Autodesk Fusion 360 part; units mm, degrees
(part 4 of 6)
sketch "mock keys" plane through (0, 0, 0) normal (0, -1, 0) x (1, 0, 0)
  line L0 (140.1031, 86.5919) -> (126.1031, 86.5919)
  line L1 (126.1031, 86.5919) -> (126.1031, 100.5919)
  line L2 (126.1031, 100.5919) -> (140.1031, 100.5919)
  line L3 (140.1031, 100.5919) -> (140.1031, 86.5919)
  line L4 (30.8531, 93.7533) -> (30.8531, 107.7533)
  line L5 (30.8531, 107.7533) -> (44.8531, 107.7533)
  line L6 (44.8531, 107.7533) -> (44.8531, 93.7533)
  line L7 (44.8531, 93.7533) -> (30.8531, 93.7533)
  line L8 (126.1031, 67.5419) -> (126.1031, 81.5419)
  line L9 (126.1031, 81.5419) -> (140.1031, 81.5419)
  line L10 (140.1031, 81.5419) -> (140.1031, 67.5419)
  line L11 (140.1031, 67.5419) -> (126.1031, 67.5419)
  line L12 (49.9031, 98.5158) -> (49.9031, 112.5158)
  line L13 (49.9031, 112.5158) -> (63.9031, 112.5158)
  line L14 (63.9031, 112.5158) -> (63.9031, 98.5158)
  line L15 (63.9031, 98.5158) -> (49.9031, 98.5158)
  line L16 (107.0531, 96.1169) -> (107.0531, 110.1169)
  line L17 (107.0531, 110.1169) -> (121.0531, 110.1169)
  line L18 (121.0531, 110.1169) -> (121.0531, 96.1169)
  line L19 (121.0531, 96.1169) -> (107.0531, 96.1169)
  line L20 (11.8031, 93.7533) -> (11.8031, 107.7533)
  line L21 (11.8031, 107.7533) -> (25.8031, 107.7533)
  line L22 (25.8031, 107.7533) -> (25.8031, 93.7533)
  line L23 (25.8031, 93.7533) -> (11.8031, 93.7533)
  line L24 (49.9031, 41.3658) -> (49.9031, 55.3658)
  line L25 (49.9031, 55.3658) -> (63.9031, 55.3658)
  line L26 (63.9031, 55.3658) -> (63.9031, 41.3658)
  line L27 (63.9031, 41.3658) -> (49.9031, 41.3658)
  line L28 (30.8531, 74.7033) -> (30.8531, 88.7033)
  line L29 (30.8531, 88.7033) -> (44.8531, 88.7033)
  line L30 (44.8531, 88.7033) -> (44.8531, 74.7033)
  line L31 (44.8531, 74.7033) -> (30.8531, 74.7033)
  line L32 (30.8531, 55.6533) -> (30.8531, 69.6533)
  line L33 (30.8531, 69.6533) -> (44.8531, 69.6533)
  line L34 (44.8531, 69.6533) -> (44.8531, 55.6533)
  line L35 (44.8531, 55.6533) -> (30.8531, 55.6533)
  line L36 (11.8031, 17.5533) -> (11.8031, 31.5533)
  line L37 (11.8031, 31.5533) -> (25.8031, 31.5533)
  line L38 (25.8031, 31.5533) -> (25.8031, 17.5533)
  line L39 (25.8031, 17.5533) -> (11.8031, 17.5533)
  line L40 (116.8975, 10.2287) -> (104.7731, 17.2287)
  line L41 (104.7731, 17.2287) -> (106.7731, 20.6928)
  line L42 (106.7731, 20.6928) -> (104.9761, 21.7303)
  line L43 (104.9761, 21.7303) -> (103.3761, 18.959)
  line L44 (103.3761, 18.959) -> (98.3098, 21.884)
  line L45 (98.3098, 21.884) -> (104.5098, 32.6227)
  line L46 (104.5098, 32.6227) -> (109.5761, 29.6977)
  line L47 (109.5761, 29.6977) -> (107.9761, 26.9264)
  line L48 (107.9761, 26.9264) -> (109.7731, 25.8889)
  line L49 (109.7731, 25.8889) -> (111.7731, 29.353)
  line L50 (111.7731, 29.353) -> (123.8975, 22.353)
  line L51 (123.8975, 22.353) -> (121.8975, 18.8889)
  line L52 (121.8975, 18.8889) -> (123.6945, 17.8514)
  line L53 (123.6945, 17.8514) -> (125.2945, 20.6227)
  line L54 (125.2945, 20.6227) -> (130.3607, 17.6977)
  line L55 (130.3607, 17.6977) -> (124.1607, 6.959)
  line L56 (124.1607, 6.959) -> (119.0945, 9.884)
  line L57 (119.0945, 9.884) -> (120.6945, 12.6553)
  line L58 (120.6945, 12.6553) -> (118.8975, 13.6928)
  line L59 (118.8975, 13.6928) -> (116.8975, 10.2287)
  line L60 (30.8531, 36.6033) -> (30.8531, 50.6033)
  line L61 (30.8531, 50.6033) -> (44.8531, 50.6033)
  line L62 (44.8531, 50.6033) -> (44.8531, 36.6033)
  line L63 (44.8531, 36.6033) -> (30.8531, 36.6033)
  line L64 (11.8031, 36.6033) -> (11.8031, 50.6033)
  line L65 (11.8031, 50.6033) -> (25.8031, 50.6033)
  line L66 (25.8031, 50.6033) -> (25.8031, 36.6033)
  line L67 (25.8031, 36.6033) -> (11.8031, 36.6033)
  line L68 (11.8031, 55.6533) -> (11.8031, 69.6533)
  line L69 (11.8031, 69.6533) -> (25.8031, 69.6533)
  line L70 (25.8031, 69.6533) -> (25.8031, 55.6533)
  line L71 (25.8031, 55.6533) -> (11.8031, 55.6533)
  line L72 (11.8031, 74.7033) -> (11.8031, 88.7033)
  line L73 (11.8031, 88.7033) -> (25.8031, 88.7033)
  line L74 (25.8031, 88.7033) -> (25.8031, 74.7033)
  line L75 (25.8031, 74.7033) -> (11.8031, 74.7033)
  line L76 (134.7127, 21.9762) -> (122.5884, 28.9762)
  line L77 (122.5884, 28.9762) -> (129.5884, 41.1005)
  line L78 (129.5884, 41.1005) -> (141.7127, 34.1005)
  line L79 (141.7127, 34.1005) -> (134.7127, 21.9762)
  line L80 (141.6977, -4.0941) -> (129.5734, 2.9059)
  line L81 (129.5734, 2.9059) -> (136.5734, 15.0302)
  line L82 (136.5734, 15.0302) -> (148.6977, 8.0302)
  line L83 (148.6977, 8.0302) -> (141.6977, -4.0941)
  line L84 (30.8531, 17.5533) -> (30.8531, 31.5533)
  line L85 (30.8531, 31.5533) -> (44.8531, 31.5533)
  line L86 (44.8531, 31.5533) -> (44.8531, 17.5533)
  line L87 (44.8531, 17.5533) -> (30.8531, 17.5533)
  line L88 (49.9031, 22.3158) -> (49.9031, 36.3158)
  line L89 (49.9031, 36.3158) -> (63.9031, 36.3158)
  line L90 (63.9031, 36.3158) -> (63.9031, 22.3158)
  line L91 (63.9031, 22.3158) -> (49.9031, 22.3158)
  line L92 (68.9531, 100.8794) -> (68.9531, 114.8794)
  line L93 (68.9531, 114.8794) -> (82.9531, 114.8794)
  line L94 (82.9531, 114.8794) -> (82.9531, 100.8794)
  line L95 (82.9531, 100.8794) -> (68.9531, 100.8794)
  line L96 (68.9531, 81.8294) -> (68.9531, 95.8294)
  line L97 (68.9531, 95.8294) -> (82.9531, 95.8294)
  line L98 (82.9531, 95.8294) -> (82.9531, 81.8294)
  line L99 (82.9531, 81.8294) -> (68.9531, 81.8294)
  line L100 (68.9531, 62.7794) -> (68.9531, 76.7794)
  line L101 (68.9531, 76.7794) -> (82.9531, 76.7794)
  line L102 (82.9531, 76.7794) -> (82.9531, 62.7794)
  line L103 (82.9531, 62.7794) -> (68.9531, 62.7794)
  line L104 (68.9531, 43.7294) -> (68.9531, 57.7294)
  line L105 (68.9531, 57.7294) -> (82.9531, 57.7294)
  line L106 (82.9531, 57.7294) -> (82.9531, 43.7294)
  line L107 (82.9531, 43.7294) -> (68.9531, 43.7294)
  line L108 (76.5731, 22.3158) -> (76.5731, 36.3158)
  line L109 (76.5731, 36.3158) -> (90.5731, 36.3158)
  line L110 (90.5731, 36.3158) -> (90.5731, 22.3158)
  line L111 (90.5731, 22.3158) -> (76.5731, 22.3158)
  line L112 (49.9031, 60.4158) -> (49.9031, 74.4158)
  line L113 (49.9031, 74.4158) -> (63.9031, 74.4158)
  line L114 (63.9031, 74.4158) -> (63.9031, 60.4158)
  line L115 (63.9031, 60.4158) -> (49.9031, 60.4158)
  line L116 (49.9031, 79.4658) -> (49.9031, 93.4658)
  line L117 (49.9031, 93.4658) -> (63.9031, 93.4658)
  line L118 (63.9031, 93.4658) -> (63.9031, 79.4658)
  line L119 (63.9031, 79.4658) -> (49.9031, 79.4658)
  line L120 (126.1031, 48.4919) -> (126.1031, 62.4919)
  line L121 (126.1031, 62.4919) -> (140.1031, 62.4919)
  line L122 (140.1031, 62.4919) -> (140.1031, 48.4919)
  line L123 (140.1031, 48.4919) -> (126.1031, 48.4919)
  line L124 (88.0031, 60.4158) -> (88.0031, 74.4158)
  line L125 (88.0031, 74.4158) -> (102.0031, 74.4158)
  line L126 (102.0031, 74.4158) -> (102.0031, 60.4158)
  line L127 (102.0031, 60.4158) -> (88.0031, 60.4158)
  line L128 (107.0531, 91.0669) -> (121.0531, 91.0669)
  line L129 (121.0531, 91.0669) -> (121.0531, 77.0669)
  line L130 (121.0531, 77.0669) -> (107.0531, 77.0669)
  line L131 (107.0531, 77.0669) -> (107.0531, 91.0669)
  line L132 (88.0031, 79.4658) -> (88.0031, 93.4658)
  line L133 (88.0031, 93.4658) -> (102.0031, 93.4658)
  line L134 (102.0031, 93.4658) -> (102.0031, 79.4658)
  line L135 (102.0031, 79.4658) -> (88.0031, 79.4658)
  line L136 (107.0531, 58.0169) -> (107.0531, 72.0169)
  line L137 (107.0531, 72.0169) -> (121.0531, 72.0169)
  line L138 (121.0531, 72.0169) -> (121.0531, 58.0169)
  line L139 (121.0531, 58.0169) -> (107.0531, 58.0169)
  line L140 (107.0531, 38.9669) -> (107.0531, 52.9669)
  line L141 (107.0531, 52.9669) -> (121.0531, 52.9669)
  line L142 (121.0531, 52.9669) -> (121.0531, 38.9669)
  line L143 (121.0531, 38.9669) -> (107.0531, 38.9669)
  line L144 (88.0031, 41.3658) -> (88.0031, 55.3658)
  line L145 (88.0031, 55.3658) -> (102.0031, 55.3658)
  line L146 (102.0031, 55.3658) -> (102.0031, 41.3658)
  line L147 (102.0031, 41.3658) -> (88.0031, 41.3658)
  circle A0 centre (71.0494, 18.8031) radius 1.1
  line L148 (102.0031, 112.5158) -> (102.0031, 98.5158)
  line L149 (102.0031, 98.5158) -> (88.0031, 98.5158)
  line L150 (88.0031, 98.5158) -> (88.0031, 112.5158)
  line L151 (88.0031, 112.5158) -> (102.0031, 112.5158)
  circle A1 centre (18.8031, 34.0783) radius 1.1
  circle A2 centre (28.3281, 91.2283) radius 1.1
  circle A3 centre (95.25, 34.2547) radius 1.1
  circle A4 centre (115.7464, 33.7256) radius 1.1
  circle A5 centre (146.7556, 76.7997) radius 1.1
  circle A6 centre (157.6917, 44.4147) radius 1.1
  circle A7 centre (146.7556, 37.8883) radius 1.1
  line L152 (151.2227, 12.4159) -> (139.0984, 19.4159)
  line L153 (139.0984, 19.4159) -> (146.0984, 31.5402)
  line L154 (146.0984, 31.5402) -> (158.2227, 24.5402)
  line L155 (158.2227, 24.5402) -> (151.2227, 12.4159)
  circle A8 centre (123.5781, 102.5878) radius 1.1
  circle A9 centre (66.4281, 78.105) radius 1.1
  circle A10 centre (130.9158, 10.2658) radius 1.1
  arc A11 (142.7339, 99.2011) -> (138.7122, 103.2228) centre (138.7122, 99.2011) ccw
  line L156 (138.7122, 103.2228) -> (132.5162, 103.2228)
  arc A12 (131.5417, 103.3426) -> (132.5162, 103.2228) centre (132.5162, 107.2444) ccw
  line L157 (131.5417, 103.3426) -> (126.6957, 104.553)
  arc A13 (123.6486, 108.4548) -> (126.6957, 104.553) centre (127.6703, 108.4548) ccw
  line L158 (123.6486, 108.4548) -> (123.6486, 112.6772)
  line L159 (123.6486, 112.6772) -> (84.9842, 117.4397)
  line L160 (84.9842, 117.4397) -> (66.9572, 117.4397)
  line L161 (66.9572, 117.4397) -> (9.2428, 110.3136)
  line L162 (9.2428, 110.3136) -> (9.2428, 14.9931)
  line L163 (9.2428, 14.9931) -> (103.8578, 14.9931)
  line L164 (103.8578, 14.9931) -> (142.6281, -7.5847)
  line L165 (142.6281, -7.5847) -> (161.7839, 25.5411)
  line L166 (161.7839, 25.5411) -> (152.8134, 30.7285)
  arc A14 (150.7772, 34.2581) -> (152.8134, 30.7285) centre (154.8544, 34.2581) ccw
  line L167 (150.7772, 34.2581) -> (150.7772, 36.2632)
  arc A15 (154.8573, 40.3375) -> (150.7772, 36.2632) centre (154.8544, 36.2603) ccw
  line L168 (154.8573, 40.3375) -> (157.6917, 40.3375)
  arc A16 (157.6917, 40.3375) -> (157.6917, 48.4919) centre (157.6917, 44.4147) ccw
  line L169 (157.6917, 48.4919) -> (146.8111, 48.4919)
  arc A17 (142.7339, 52.5692) -> (146.8111, 48.4919) centre (146.8111, 52.5692) ccw
  line L170 (142.7339, 52.5692) -> (142.7339, 68.7564)
  arc A18 (146.7556, 72.7781) -> (142.7339, 68.7564) centre (146.7556, 68.7564) ccw
  arc A19 (146.7556, 72.7781) -> (146.7556, 80.8214) centre (146.7556, 76.7997) ccw
  arc A20 (142.7339, 84.843) -> (146.7556, 80.8214) centre (146.7556, 84.843) ccw
  line L171 (142.7339, 84.843) -> (142.7339, 99.2011)
  line L172 (9.8031, 71.6533) -> (27.8031, 71.6533)
  line L173 (27.8031, 71.6533) -> (27.8031, 53.6533)
  line L174 (27.8031, 53.6533) -> (9.8031, 53.6533)
  line L175 (9.8031, 53.6533) -> (9.8031, 71.6533)
  line L176 (9.8031, 91.7533) -> (9.8031, 109.7533)
  line L177 (27.8031, 91.7533) -> (9.8031, 91.7533)
  line L178 (9.8031, 109.7533) -> (27.8031, 109.7533)
  line L179 (27.8031, 109.7533) -> (27.8031, 91.7533)
  line L180 (9.8031, 15.5533) -> (9.8031, 33.5533)
  line L181 (27.8031, 15.5533) -> (9.8031, 15.5533)
  line L182 (9.8031, 33.5533) -> (27.8031, 33.5533)
  line L183 (27.8031, 33.5533) -> (27.8031, 15.5533)
  line L184 (9.8031, 34.6033) -> (9.8031, 52.6033)
  line L185 (27.8031, 34.6033) -> (9.8031, 34.6033)
  line L186 (9.8031, 52.6033) -> (27.8031, 52.6033)
  line L187 (27.8031, 52.6033) -> (27.8031, 34.6033)
  line L188 (124.1031, 84.5919) -> (124.1031, 102.5919)
  line L189 (142.1031, 84.5919) -> (124.1031, 84.5919)
  line L190 (124.1031, 102.5919) -> (142.1031, 102.5919)
  line L191 (142.1031, 102.5919) -> (142.1031, 84.5919)
  line L192 (124.1031, 65.5419) -> (124.1031, 83.5419)
  line L193 (142.1031, 65.5419) -> (124.1031, 65.5419)
  line L194 (124.1031, 83.5419) -> (142.1031, 83.5419)
  line L195 (142.1031, 83.5419) -> (142.1031, 65.5419)
  line L196 (124.1031, 46.4919) -> (124.1031, 64.4919)
  line L197 (142.1031, 46.4919) -> (124.1031, 46.4919)
  line L198 (124.1031, 64.4919) -> (142.1031, 64.4919)
  line L199 (142.1031, 64.4919) -> (142.1031, 46.4919)
  line L200 (9.8031, 72.7033) -> (9.8031, 90.7033)
  line L201 (27.8031, 72.7033) -> (9.8031, 72.7033)
  line L202 (9.8031, 90.7033) -> (27.8031, 90.7033)
  line L203 (27.8031, 90.7033) -> (27.8031, 72.7033)
  line L204 (25.8031, 17.5533) -> (25.8031, 31.5533)
  line L205 (11.8031, 31.5533) -> (11.8031, 17.5533)
  line L206 (25.8031, 31.5533) -> (11.8031, 31.5533)
  line L207 (11.8031, 17.5533) -> (25.8031, 17.5533)
  line L208 (30.8531, 17.5533) -> (44.8531, 17.5533)
  line L209 (30.8531, 31.5533) -> (30.8531, 17.5533)
  line L210 (44.8531, 31.5533) -> (30.8531, 31.5533)
  line L211 (44.8531, 17.5533) -> (44.8531, 31.5533)
  line L212 (90.3624, 253.2917) -> (90.3624, 271.2917)
  line L213 (90.3624, 195.0917) -> (108.3624, 195.0917)
  line L214 (90.3624, 252.2417) -> (108.3624, 252.2417)
  line L215 (108.3624, 214.1417) -> (108.3624, 196.1417)
  line L216 (90.3624, 215.1917) -> (90.3624, 233.1917)
  line L217 (108.3624, 196.1417) -> (90.3624, 196.1417)
  line L218 (90.3624, 214.1417) -> (108.3624, 214.1417)
  line L219 (90.3624, 177.0917) -> (90.3624, 195.0917)
  line L220 (108.3624, 234.2417) -> (90.3624, 234.2417)
  line L221 (108.3624, 271.2917) -> (108.3624, 253.2917)
  line L222 (108.3624, 215.1917) -> (90.3624, 215.1917)
  line L223 (108.3624, 253.2917) -> (90.3624, 253.2917)
  line L224 (90.3624, 234.2417) -> (90.3624, 252.2417)
  line L225 (90.3624, 196.1417) -> (90.3624, 214.1417)
  line L226 (108.3624, 233.1917) -> (108.3624, 215.1917)
  line L227 (90.3624, 271.2917) -> (108.3624, 271.2917)
  line L228 (108.3624, 177.0917) -> (90.3624, 177.0917)
  line L229 (90.3624, 233.1917) -> (108.3624, 233.1917)
  line L230 (108.3624, 252.2417) -> (108.3624, 234.2417)
  line L231 (108.3624, 195.0917) -> (108.3624, 177.0917)
  line L232 (90.3624, 195.0917) -> (108.3624, 195.0917)
  line L233 (90.3624, 177.0917) -> (90.3624, 195.0917)
  line L234 (108.3624, 195.0917) -> (108.3624, 177.0917)
  line L235 (108.3624, 252.2417) -> (108.3624, 234.2417)
  line L236 (108.3624, 214.1417) -> (108.3624, 196.1417)
  line L237 (90.3624, 253.2917) -> (90.3624, 271.2917)
  line L238 (90.3624, 196.1417) -> (90.3624, 214.1417)
  line L239 (90.3624, 215.1917) -> (90.3624, 233.1917)
  line L240 (108.3624, 233.1917) -> (108.3624, 215.1917)
  line L241 (108.3624, 271.2917) -> (108.3624, 253.2917)
  line L242 (90.3624, 234.2417) -> (90.3624, 252.2417)
  line L243 (90.3624, 233.1917) -> (108.3624, 233.1917)
  line L244 (108.3624, 253.2917) -> (90.3624, 253.2917)
  line L245 (90.3624, 214.1417) -> (108.3624, 214.1417)
  line L246 (108.3624, 177.0917) -> (90.3624, 177.0917)
  line L247 (108.3624, 215.1917) -> (90.3624, 215.1917)
  line L248 (90.3624, 252.2417) -> (108.3624, 252.2417)
  line L249 (108.3624, 234.2417) -> (90.3624, 234.2417)
  line L250 (108.3624, 196.1417) -> (90.3624, 196.1417)
  line L251 (90.3624, 271.2917) -> (108.3624, 271.2917)
  line L252 (28.8531, 33.5533) -> (46.8531, 33.5533)
  line L253 (28.8531, 15.5533) -> (28.8531, 33.5533)
  line L254 (46.8531, 33.5533) -> (46.8531, 15.5533)
  line L255 (46.8531, 90.7033) -> (46.8531, 72.7033)
  line L256 (46.8531, 52.6033) -> (46.8531, 34.6033)
  line L257 (28.8531, 91.7533) -> (28.8531, 109.7533)
  line L258 (28.8531, 34.6033) -> (28.8531, 52.6033)
  line L259 (28.8531, 53.6533) -> (28.8531, 71.6533)
  line L260 (46.8531, 71.6533) -> (46.8531, 53.6533)
  line L261 (46.8531, 109.7533) -> (46.8531, 91.7533)
  line L262 (28.8531, 72.7033) -> (28.8531, 90.7033)
  line L263 (28.8531, 71.6533) -> (46.8531, 71.6533)
  line L264 (46.8531, 91.7533) -> (28.8531, 91.7533)
  line L265 (28.8531, 52.6033) -> (46.8531, 52.6033)
  line L266 (46.8531, 15.5533) -> (28.8531, 15.5533)
  line L267 (46.8531, 53.6533) -> (28.8531, 53.6533)
  line L268 (28.8531, 90.7033) -> (46.8531, 90.7033)
  line L269 (46.8531, 72.7033) -> (28.8531, 72.7033)
  line L270 (46.8531, 34.6033) -> (28.8531, 34.6033)
  line L271 (28.8531, 109.7533) -> (46.8531, 109.7533)
  line L272 (47.9031, 38.3158) -> (65.9031, 38.3158)
  line L273 (47.9031, 20.3158) -> (47.9031, 38.3158)
  line L274 (65.9031, 38.3158) -> (65.9031, 20.3158)
  line L275 (65.9031, 95.4658) -> (65.9031, 77.4658)
  line L276 (65.9031, 57.3658) -> (65.9031, 39.3658)
  line L277 (47.9031, 96.5158) -> (47.9031, 114.5158)
  line L278 (47.9031, 39.3658) -> (47.9031, 57.3658)
  line L279 (47.9031, 58.4158) -> (47.9031, 76.4158)
  line L280 (65.9031, 76.4158) -> (65.9031, 58.4158)
  line L281 (65.9031, 114.5158) -> (65.9031, 96.5158)
  line L282 (47.9031, 77.4658) -> (47.9031, 95.4658)
  line L283 (47.9031, 76.4158) -> (65.9031, 76.4158)
  line L284 (65.9031, 96.5158) -> (47.9031, 96.5158)
  line L285 (47.9031, 57.3658) -> (65.9031, 57.3658)
  line L286 (65.9031, 20.3158) -> (47.9031, 20.3158)
  line L287 (65.9031, 58.4158) -> (47.9031, 58.4158)
  line L288 (47.9031, 95.4658) -> (65.9031, 95.4658)
  line L289 (65.9031, 77.4658) -> (47.9031, 77.4658)
  line L290 (65.9031, 39.3658) -> (47.9031, 39.3658)
  line L291 (47.9031, 114.5158) -> (65.9031, 114.5158)
  line L292 (84.9531, 97.8294) -> (84.9531, 79.8294)
  line L293 (84.9531, 59.7294) -> (84.9531, 41.7294)
  line L294 (66.9531, 98.8794) -> (66.9531, 116.8794)
  line L295 (66.9531, 41.7294) -> (66.9531, 59.7294)
  line L296 (66.9531, 60.7794) -> (66.9531, 78.7794)
  line L297 (84.9531, 78.7794) -> (84.9531, 60.7794)
  line L298 (84.9531, 116.8794) -> (84.9531, 98.8794)
  line L299 (66.9531, 79.8294) -> (66.9531, 97.8294)
  line L300 (66.9531, 78.7794) -> (84.9531, 78.7794)
  line L301 (84.9531, 98.8794) -> (66.9531, 98.8794)
  line L302 (66.9531, 59.7294) -> (84.9531, 59.7294)
  line L303 (84.9531, 60.7794) -> (66.9531, 60.7794)
  line L304 (66.9531, 97.8294) -> (84.9531, 97.8294)
  line L305 (84.9531, 79.8294) -> (66.9531, 79.8294)
  line L306 (84.9531, 41.7294) -> (66.9531, 41.7294)
  line L307 (66.9531, 116.8794) -> (84.9531, 116.8794)
  line L308 (104.0031, 95.4658) -> (104.0031, 77.4658)
  line L309 (104.0031, 57.3658) -> (104.0031, 39.3658)
  line L310 (86.0031, 96.5158) -> (86.0031, 114.5158)
  line L311 (86.0031, 39.3658) -> (86.0031, 57.3658)
  line L312 (86.0031, 58.4158) -> (86.0031, 76.4158)
  line L313 (104.0031, 76.4158) -> (104.0031, 58.4158)
  line L314 (104.0031, 114.5158) -> (104.0031, 96.5158)
  line L315 (86.0031, 77.4658) -> (86.0031, 95.4658)
  line L316 (86.0031, 76.4158) -> (104.0031, 76.4158)
  line L317 (104.0031, 96.5158) -> (86.0031, 96.5158)
  line L318 (86.0031, 57.3658) -> (104.0031, 57.3658)
  line L319 (104.0031, 58.4158) -> (86.0031, 58.4158)
  line L320 (86.0031, 95.4658) -> (104.0031, 95.4658)
  line L321 (104.0031, 77.4658) -> (86.0031, 77.4658)
  line L322 (104.0031, 39.3658) -> (86.0031, 39.3658)
  line L323 (86.0031, 114.5158) -> (104.0031, 114.5158)
  line L324 (123.0531, 93.0669) -> (123.0531, 75.0669)
  line L325 (123.0531, 54.9669) -> (123.0531, 36.9669)
  line L326 (105.0531, 94.1169) -> (105.0531, 112.1169)
  line L327 (105.0531, 36.9669) -> (105.0531, 54.9669)
  line L328 (105.0531, 56.0169) -> (105.0531, 74.0169)
  line L329 (123.0531, 74.0169) -> (123.0531, 56.0169)
  line L330 (123.0531, 112.1169) -> (123.0531, 94.1169)
  line L331 (105.0531, 75.0669) -> (105.0531, 93.0669)
  line L332 (105.0531, 74.0169) -> (123.0531, 74.0169)
  line L333 (123.0531, 94.1169) -> (105.0531, 94.1169)
  line L334 (105.0531, 54.9669) -> (123.0531, 54.9669)
  line L335 (123.0531, 56.0169) -> (105.0531, 56.0169)
  line L336 (105.0531, 93.0669) -> (123.0531, 93.0669)
  line L337 (123.0531, 75.0669) -> (105.0531, 75.0669)
  line L338 (123.0531, 36.9669) -> (105.0531, 36.9669)
  line L339 (105.0531, 112.1169) -> (123.0531, 112.1169)
  line L340 (74.5731, 38.3158) -> (92.5731, 38.3158)
  line L341 (92.5731, 38.3158) -> (92.5731, 20.3158)
  line L342 (92.5731, 20.3158) -> (74.5731, 20.3158)
  line L343 (74.5731, 20.3158) -> (74.5731, 38.3158)
  line L344 (94.2468, 20.9966) -> (103.2468, 36.5851)
  line L345 (103.2468, 36.5851) -> (134.4237, 18.5851)
  line L346 (134.4237, 18.5851) -> (125.4237, 2.9966)
  line L347 (125.4237, 2.9966) -> (94.2468, 20.9966)
  line L348 (119.8563, 28.2441) -> (128.8563, 43.8326)
  line L349 (128.8563, 43.8326) -> (144.4448, 34.8326)
  line L350 (144.4448, 34.8326) -> (135.4448, 19.2441)
  line L351 (135.4448, 19.2441) -> (119.8563, 28.2441)
  line L352 (145.3663, 34.2723) -> (160.9548, 25.2723)
  line L353 (160.9548, 25.2723) -> (151.9548, 9.6838)
  line L354 (136.3663, 18.6838) -> (145.3663, 34.2723)
  line L355 (151.9548, 9.6838) -> (136.3663, 18.6838)
  line L356 (135.8413, 17.7623) -> (151.4298, 8.7623)
  line L357 (151.4298, 8.7623) -> (142.4298, -6.8262)
  line L358 (126.8413, 2.1738) -> (135.8413, 17.7623)
  line L359 (142.4298, -6.8262) -> (126.8413, 2.1738)
  dimension "d350" = 18
  dimension "d351" = 18
  dimension "d352" = 18
  dimension "d353" = 18
  dimension "d354" = 18
  dimension "d355" = 18
  dimension "d356" = 18
  dimension "d357" = 18
  dimension "d358" = 18
  dimension "d359" = 18
  dimension "d360" = 18
  dimension "d361" = 18
  dimension "d362" = 18
  dimension "d363" = 18
  dimension "d364" = 18
  dimension "d365" = 18
  dimension "d366" = 2
  dimension "d367" = 2
  dimension "d368" = 2
  dimension "d369" = 2
  dimension "d370" = 2
  dimension "d371" = 2
  dimension "d372" = 2
  dimension "d373" = 2
  dimension "d374" = 2
  dimension "d375" = 2
  dimension "d376" = 2
  dimension "d377" = 2
  dimension "d378" = 2
  dimension "d379" = 2
  dimension "d380" = 2
  dimension "d381" = 2
  dimension "d420" = 18
  dimension "d421" = 18
  dimension "d422" = 18
  dimension "d423" = 18
  dimension "d426" = 18
  dimension "d427" = 18
  dimension "d428" = 18
  dimension "d429" = 18
  dimension "d434" = 18
  dimension "d435" = 18
  dimension "d436" = 1.05
  dimension "d437" = 1.05
  dimension "d440" = 1.05
  dimension "d441" = 1.05
  dimension "d442" = 18
  dimension "d443" = 18
  dimension "d444" = 18
  dimension "d445" = 18
  dimension "d446" = 18
  dimension "d447" = 18
  dimension "d448" = 18
  dimension "d449" = 18
  dimension "d450" = 18
  dimension "d451" = 18
  dimension "d452" = 1.05
  dimension "d453" = 1.05
  dimension "d454" = 1.05
  dimension "d455" = 1.05
  dimension "d456" = 18
  dimension "d457" = 18
  dimension "d458" = 18
  dimension "d459" = 18
  dimension "d460" = 18
  dimension "d461" = 18
  dimension "d462" = 18
  dimension "d463" = 18
  dimension "d464" = 18
  dimension "d465" = 18
  dimension "d466" = 1.05
  dimension "d467" = 1.05
  dimension "d468" = 1.05
  dimension "d469" = 1.05
  dimension "d470" = 2
  dimension "d471" = 2
  dimension "d472" = 18
  dimension "d473" = 18
  dimension "d474" = 18
  dimension "d475" = 18
  dimension "d476" = 18
  dimension "d477" = 18
  dimension "d478" = 18
  dimension "d479" = 18
  dimension "d480" = 18
  dimension "d481" = 18
  dimension "d482" = 1.05
  dimension "d483" = 1.05
  dimension "d484" = 1.05
  dimension "d485" = 1.05
  dimension "d486" = 2
  dimension "d487" = 2
  dimension "d490" = 18
  dimension "d491" = 18
  dimension "d492" = 18
  dimension "d493" = 18
  dimension "d494" = 18
  dimension "d495" = 18
  dimension "d496" = 18
  dimension "d497" = 18
  dimension "d499" = 1.05
  dimension "d500" = 1.05
  dimension "d501" = 1.05
  dimension "d502" = 2
  dimension "d503" = 2
  dimension "d506" = 18
  dimension "d507" = 18
  dimension "d508" = 18
  dimension "d509" = 18
  dimension "d510" = 18
  dimension "d511" = 18
  dimension "d512" = 18
  dimension "d513" = 18
  dimension "d515" = 1.05
  dimension "d516" = 1.05
  dimension "d517" = 1.05
  dimension "d518" = 2
  dimension "d519" = 2
  dimension "d522" = 18
  dimension "d523" = 18
  dimension "d524" = 18
  dimension "d525" = 18
  dimension "d526" = 18
  dimension "d527" = 18
  dimension "d528" = 18
  dimension "d529" = 18
  dimension "d531" = 1.05
  dimension "d532" = 1.05
  dimension "d533" = 1.05
  dimension "d535" = 2
  dimension "d536" = 2
  dimension "d537" = 18
  dimension "d538" = 18
  dimension "d539" = 2
  dimension "d540" = 2
  dimension "d541" = 18
  dimension "d542" = 18
  dimension "d543" = 2
  dimension "d544" = 2
  dimension "d545" = 3.075
  dimension "d546" = 2
  dimension "d547" = 18
  dimension "d548" = 36
  dimension "d549" = 3.075
  dimension "d550" = 18
  dimension "d551" = 18
  dimension "d552" = 18
  dimension "d553" = 18
  dimension "d554" = 2
  dimension "d555" = 2
  dimension "d556" = 2
  dimension "d557" = 2
  constraint horizontal L172
  constraint vertical L173
  constraint horizontal L174
  constraint vertical L175
  constraint horizontal L178
  constraint vertical L179
  constraint horizontal L177
  constraint vertical L176
  constraint horizontal L182
  constraint vertical L183
  constraint horizontal L181
  constraint vertical L180
  constraint horizontal L186
  constraint vertical L187
  constraint horizontal L185
  constraint vertical L184
  constraint horizontal L190
  constraint vertical L191
  constraint horizontal L189
  constraint vertical L188
  constraint horizontal L194
  constraint vertical L195
  constraint horizontal L193
  constraint vertical L192
  constraint horizontal L198
  constraint vertical L199
  constraint horizontal L197
  constraint vertical L196
  constraint horizontal L202
  constraint vertical L203
  constraint horizontal L201
  constraint vertical L200
  constraint horizontal L213
  constraint vertical L231
  constraint horizontal L228
  constraint vertical L219
  constraint horizontal L218
  constraint vertical L215
  constraint horizontal L217
  constraint vertical L225
  constraint horizontal L229
  constraint vertical L226
  constraint horizontal L222
  constraint vertical L216
  constraint horizontal L227
  constraint vertical L221
  constraint horizontal L223
  constraint vertical L212
  constraint horizontal L214
  constraint vertical L230
  constraint horizontal L220
  constraint vertical L224
  constraint collinear L216 L224
  constraint collinear L219 L225
  constraint collinear L221 L230
  constraint collinear L215 L226
  constraint horizontal L232
  constraint vertical L234
  constraint horizontal L246
  constraint vertical L233
  constraint horizontal L245
  constraint vertical L236
  constraint horizontal L250
  constraint vertical L238
  constraint horizontal L243
  constraint vertical L240
  constraint horizontal L247
  constraint vertical L239
  constraint horizontal L251
  constraint vertical L241
  constraint horizontal L244
  constraint vertical L237
  constraint horizontal L248
  constraint vertical L235
  constraint horizontal L249
  constraint vertical L242
  constraint collinear L239 L242
  constraint collinear L233 L238
  constraint collinear L235 L241
  constraint collinear L236 L240
  constraint horizontal L252
  constraint vertical L254
  constraint horizontal L266
  constraint vertical L253
  constraint horizontal L265
  constraint vertical L256
  constraint horizontal L270
  constraint vertical L258
  constraint horizontal L263
  constraint vertical L260
  constraint horizontal L267
  constraint vertical L259
  constraint horizontal L271
  constraint vertical L261
  constraint horizontal L264
  constraint vertical L257
  constraint horizontal L268
  constraint vertical L255
  constraint horizontal L269
  constraint vertical L262
  constraint collinear L259 L262
  constraint collinear L253 L258
  constraint collinear L255 L261
  constraint collinear L256 L260
  constraint horizontal L272
  constraint vertical L274
  constraint horizontal L286
  constraint vertical L273
  constraint horizontal L285
  constraint vertical L276
  constraint horizontal L290
  constraint vertical L278
  constraint horizontal L283
  constraint vertical L280
  constraint horizontal L287
  constraint vertical L279
  constraint horizontal L291
  constraint vertical L281
  constraint horizontal L284
  constraint vertical L277
  constraint horizontal L288
  constraint vertical L275
  constraint horizontal L289
  constraint vertical L282
  constraint collinear L279 L282
  constraint collinear L273 L278
  constraint collinear L275 L281
  constraint collinear L276 L280
  constraint horizontal L302
  constraint vertical L293
  constraint horizontal L306
  constraint vertical L295
  constraint horizontal L300
  constraint vertical L297
  constraint horizontal L303
  constraint vertical L296
  constraint horizontal L307
  constraint vertical L298
  constraint horizontal L301
  constraint vertical L294
  constraint horizontal L304
  constraint vertical L292
  constraint horizontal L305
  constraint vertical L299
  constraint collinear L296 L299
  constraint collinear L292 L298
  constraint collinear L293 L297
  constraint horizontal L318
  constraint vertical L309
  constraint horizontal L322
  constraint vertical L311
  constraint horizontal L316
  constraint vertical L313
  constraint horizontal L319
  constraint vertical L312
  constraint horizontal L323
  constraint vertical L314
  constraint horizontal L317
  constraint vertical L310
  constraint horizontal L320
  constraint vertical L308
  constraint horizontal L321
  constraint vertical L315
  constraint collinear L312 L315
  constraint collinear L308 L314
  constraint collinear L309 L313
  constraint horizontal L334
  constraint vertical L325
  constraint horizontal L338
  constraint vertical L327
  constraint horizontal L332
  constraint vertical L329
  constraint horizontal L335
  constraint vertical L328
  constraint horizontal L339
  constraint vertical L330
  constraint horizontal L333
  constraint vertical L326
  constraint horizontal L336
  constraint vertical L324
  constraint horizontal L337
  constraint vertical L331
  constraint collinear L328 L331
  constraint collinear L324 L330
  constraint collinear L325 L329
  constraint horizontal L340
  constraint vertical L341
  constraint horizontal L342
  constraint vertical L343
  constraint perpendicular L345 L346
  constraint perpendicular L348 L349
  constraint perpendicular L350 L351
  constraint perpendicular L346 L347
  constraint perpendicular L344 L347
  constraint perpendicular L348 L351
  constraint parallel L76 L351
  constraint parallel L50 L345
  constraint perpendicular L352 L354
  constraint perpendicular L353 L355
  constraint perpendicular L354 L355
  constraint perpendicular L356 L358
  constraint perpendicular L357 L359
  constraint perpendicular L358 L359
  measures "d350" distance of L172.start L172.end
  measures "d351" distance of L172.start L174.end
  measures "d352" distance of L178.end L176.end
  measures "d353" distance of L176.end L176.start
  measures "d354" distance of L182.end L180.end
  measures "d355" distance of L180.end L180.start
  measures "d356" distance of L186.end L184.end
  measures "d357" distance of L184.end L184.start
  measures "d358" distance of L190.end L188.end
  measures "d359" distance of L188.end L188.start
  measures "d360" distance of L194.end L192.end
  measures "d361" distance of L192.end L192.start
  measures "d362" distance of L198.end L196.end
  measures "d363" distance of L196.end L196.start
  measures "d364" distance of L202.end L200.end
  measures "d365" distance of L200.end L200.start
  measures "d366" distance of L36 L180
  measures "d367" distance of L181 L207
  measures "d368" distance of L64 L184
  measures "d369" distance of L65 L186
  measures "d370" distance of L68 L175
  measures "d371" distance of L71 L174
  measures "d372" distance of L74 L203
  measures "d373" distance of L73 L202
  measures "d374" distance of L20 L176
  measures "d375" distance of L21 L178
  measures "d376" distance of L120 L196
  measures "d377" distance of L123 L197
  measures "d378" distance of L8 L192
  measures "d379" distance of L11 L193
  measures "d380" distance of L1 L188
  measures "d381" distance of L0 L189
  measures "d420" distance of L213.start L213.end
  measures "d421" distance of L213.start L219.start
  measures "d422" distance of L218.start L215.start
  measures "d423" distance of L217.end L218.start
  measures "d426" distance of L216.end L226.start
  measures "d427" distance of L216.end L216.start
  measures "d428" distance of L212.end L221.start
  measures "d429" distance of L212.end L212.start
  measures "d434" distance of L214.end L214.start
  measures "d435" distance of L214.start L220.end
  measures "d436" distance of L213 L217
  measures "d437" distance of L218 L222
  measures "d440" distance of L220 L229
  measures "d441" distance of L214 L223
  measures "d442" distance of L213.end L213.start
  measures "d443" distance of L219.start L213.start
  measures "d444" distance of L215.start L218.start
  measures "d445" distance of L218.start L217.end
  measures "d446" distance of L216.end L226.start
  measures "d447" distance of L216.end L216.start
  measures "d448" distance of L212.end L221.start
  measures "d449" distance of L212.end L212.start
  measures "d450" distance of L214.start L214.end
  measures "d451" distance of L214.start L220.end
  measures "d452" distance of L232 L250
  measures "d453" distance of L245 L247
  measures "d454" distance of L243 L249
  measures "d455" distance of L244 L248
  measures "d456" distance of L252.end L252.start
  measures "d457" distance of L253.start L252.start
  measures "d458" distance of L256.start L258.end
  measures "d459" distance of L258.end L258.start
  measures "d460" distance of L259.end L260.start
  measures "d461" distance of L259.end L259.start
  measures "d462" distance of L257.end L261.start
  measures "d463" distance of L257.end L257.start
  measures "d464" distance of L262.end L255.start
  measures "d465" distance of L262.end L262.start
  measures "d466" distance of L252 L270
  measures "d467" distance of L265 L267
  measures "d468" distance of L263 L269
  measures "d469" distance of L264 L268
  measures "d470" distance of L5 L271
  measures "d471" distance of L34 L260
  measures "d472" distance of L272.end L272.start
  measures "d473" distance of L273.start L272.start
  measures "d474" distance of L276.start L278.end
  measures "d475" distance of L278.end L278.start
  measures "d476" distance of L279.end L280.start
  measures "d477" distance of L279.end L279.start
  measures "d478" distance of L277.end L281.start
  measures "d479" distance of L277.end L277.start
  measures "d480" distance of L282.end L275.start
  measures "d481" distance of L282.end L282.start
  measures "d482" distance of L272 L290
  measures "d483" distance of L285 L287
  measures "d484" distance of L283 L289
  measures "d485" distance of L284 L288
  measures "d486" distance of L14 L281
  measures "d487" distance of L13 L291
  measures "d490" distance of L293.start L295.end
  measures "d491" distance of L295.end L295.start
  measures "d492" distance of L296.end L297.start
  measures "d493" distance of L296.end L296.start
  measures "d494" distance of L294.end L298.start
  measures "d495" distance of L294.end L294.start
  measures "d496" distance of L299.end L292.start
  measures "d497" distance of L299.end L299.start
  measures "d499" distance of L302 L303
  measures "d500" distance of L300 L305
  measures "d501" distance of L301 L304
  measures "d502" distance of L94 L298
  measures "d503" distance of L93 L307
  measures "d506" distance of L309.start L311.end
  measures "d507" distance of L311.end L311.start
  measures "d508" distance of L312.end L313.start
  measures "d509" distance of L312.end L312.start
  measures "d510" distance of L310.end L314.start
  measures "d511" distance of L310.end L310.start
  measures "d512" distance of L315.end L308.start
  measures "d513" distance of L315.end L315.start
  measures "d515" distance of L318 L319
  measures "d516" distance of L316 L321
  measures "d517" distance of L317 L320
  measures "d518" distance of L148 L314
  measures "d519" distance of L151 L323
  measures "d522" distance of L325.start L327.end
  measures "d523" distance of L327.end L327.start
  measures "d524" distance of L328.end L329.start
  measures "d525" distance of L328.end L328.start
  measures "d526" distance of L326.end L330.start
  measures "d527" distance of L326.end L326.start
  measures "d528" distance of L331.end L324.start
  measures "d529" distance of L331.end L331.start
  measures "d531" distance of L334 L335
  measures "d532" distance of L332 L337
  measures "d533" distance of L333 L336
  measures "d535" distance of L17 L339
  measures "d536" distance of L142 L325
  measures "d537" distance of L340.start L340.end
  measures "d538" distance of L340.start L342.end
  measures "d539" distance of L108 L343
  measures "d540" distance of L111 L342
  measures "d541" distance of L348.start L350.end
  measures "d542" distance of L349.end L350.end
  measures "d543" distance of L77 L348
  measures "d544" distance of L78 L349
  measures "d545" distance of L45 L344
  measures "d546" distance of L50 L345
  measures "d547" distance of L345.end L346.end
  measures "d548" distance of L344.start L346.end
  measures "d549" distance of L55 L346
  measures "d550" distance of L353.end L354.start
  measures "d551" distance of L353.end L352.end
  measures "d552" distance of L357.end L358.start
  measures "d553" distance of L357.end L356.end
  measures "d554" distance of L83 L357
  measures "d555" distance of L80 L359
  measures "d556" distance of L154 L352
  measures "d557" distance of L155 L353
extrude "Extrude8" add sketch "mock keys" against normal blind 4 from surface at 9.7 separate body contours L0 L1 L2 L3 | L4 L5 L6 L7 | L8 L9 L10 L11 | L12 L13 L14 L15 | L16 L17 L18 L19 | L20 L21 L22 L23 | L24 L25 L26 L27 | L28 L29 L30 L31 | L32 L33 L34 L35 | L36 L37 L38 L39 L204 L205 L206 L207 | L40 L41 L42 L43 L44 L45 L46 L47 L48 L49 L50 L51 L52 L53 L54 L55 L56 L57 L58 L59 | L60 L61 L62 L63 | L64 L65 L66 L67 | L68 L69 L70 L71 | L72 L73 L74 L75 | L76 L77 L78 L79 | L80 L81 L82 L83 | L84 L85 L86 L87 L208 L209 L210 L211 | L88 L89 L90 L91 | L92 L93 L94 L95 | L96 L97 L98 L99 | L100 L101 L102 L103 | L104 L105 L106 L107 | L108 L109 L110 L111 | L112 L113 L114 L115 | L116 L117 L118 L119 | L120 L121 L122 L123 | L124 L125 L126 L127 | L128 L129 L130 L131 | L132 L133 L134 L135 | L136 L137 L138 L139 | L140 L141 L142 L143 | L144 L145 L146 L147 | L148 L149 L150 L151 | A1 L185 | A1 L184 L185 L186 L187 | A1 L180 L181 L182 L183 | A1 L182 | A2 L257 L264 | A2 L257 L261 L264 L271 | A2 L255 L262 L268 L269 | A2 L262 L268 | A2 L177 L179 | A2 L176 L177 L178 L179 | A2 L200 L201 L202 L203 | A2 L202 L203 | L152 L153 L154 L155 | A8 L188 L190 | A8 A11 L188 L189 L190 L191 | A8 L330 | A8 L326 L330 L333 L339 | A11 L190 L191 | A9 L296 L300 | A9 L296 L297 L300 L303 | A9 L275 L289 | A9 L275 L282 L288 L289 | A10 L358 | A10 L356 L357 L358 L359 | L172 L173 L174 L175 | L192 L193 L194 L195 | L196 L197 L198 L199 | L252 L253 L254 L266 | L256 L258 L265 L270 | L259 L260 L263 L267 | L272 L273 L274 L286 | L276 L278 L285 L290 | L277 L281 L284 L291 | L279 L280 L283 L287 | L292 L299 L304 L305 | L293 L295 L302 L306 | L294 L298 L301 L307 | L308 L315 L320 L321 | L309 L311 L318 L322 | L310 L314 L317 L323 | L312 L313 L316 L319 | L324 L331 L336 L337 | L325 L327 L334 L338 | L328 L329 L332 L335 | L340 L341 L342 L343 | L344 L345 L346 L347 | L348 L349 L350 L351 | L352 L353 L354 L355 picked at (131.7031, 9.9672) makes body 8 at (128.0525, -9.7, 30.4403) makes body 9 at (34.8531, -9.7, 27.5533) makes body 10 at (53.9031, -9.7, 45.3658) makes body 11 at (130.1031, -9.7, 58.4919) makes body 12 at (53.9031, -9.7, 70.4158) makes body 13 at (34.8531, -9.7, 78.7033) makes body 14 at (111.0531, -9.7, 81.0669) makes body 15 at (92.0031, -9.7, 102.5158) makes body 16 at (21.8031, -9.7, 97.7533) makes body 17 at (78.9531, -9.7, 110.8794) makes body 18 at (130.1031, -9.7, 71.5419) makes body 19 at (53.9031, -9.7, 83.4658) makes body 20 at (34.8531, -9.7, 65.6533) makes body 21 at (111.0531, -9.7, 68.0169) makes body 22 at (72.9531, -9.7, 47.7294) makes body 23 at (15.8031, -9.7, 27.5533) makes body 24 at (118.0314, -9.7, 14.1928) makes body 25 at (152.7586, -9.7, 23.0761) makes body 26 at (53.9031, -9.7, 32.3158) makes body 27 at (34.8531, -9.7, 40.6033) makes body 28 at (111.0531, -9.7, 42.9669) makes body 29 at (72.9531, -9.7, 72.7794) makes body 30 at (15.8031, -9.7, 84.7033) makes body 31 at (92.0031, -9.7, 83.4658) makes body 32 at (117.0531, -9.7, 106.1169) makes body 33 at (34.8531, -9.7, 103.7533) makes body 34 at (53.9031, -9.7, 102.5158) makes body 35 at (130.1031, -9.7, 90.5919) makes body 36 at (72.9531, -9.7, 85.8294) makes body 37 at (21.8031, -9.7, 59.6533) makes body 38 at (92.0031, -9.7, 70.4158) makes body 39 at (92.0031, -9.7, 45.3658) makes body 40 at (21.8031, -9.7, 40.6033) makes body 41 at (80.5731, -9.7, 32.3158) makes body 42 at (135.0375, -9.7, 4.37)
extrude "Extrude9" add sketch "wrist rest" against normal blind 6.35 from surface at 6.2 separate body makes body 43
copy_body "Body->Comp1" bodies 1 removing the originals makes body 44 in component "top plate"
copy_body "Body->Comp2" bodies 4 removing the originals makes body 45 in component "baseplate"
copy_body "Body->Comp3" bodies 7 removing the originals makes body 46 in component "battery plate"